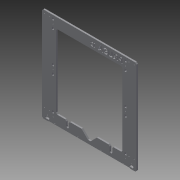
# Autodesk Inventor part: Main_frame_import
Saved by Autodesk Inventor 2015 (Build 190159000, 159)
## iProperties
Created: 2015-04-20
Part Number: Main_frame_import
Material: Generic
Document SubType Name: Modeling
Designer: X
Density: 1 g/cm^3
Appearance: Default
Author: X
Autodesk Inventor part; units mm, degrees
(part 1 of 2)
ref_plane "YZ Plane" through (0, 0, 0) normal (1, 0, 0) x (0, 1, 0)
ref_plane "XZ Plane" through (0, 0, 0) normal (0, 1, 0) x (-1, 0, 0)
ref_plane "XY Plane" through (0, 0, 0) normal (0, 0, 1) x (1, 0, 0)
sketch "Sketch1" plane through (0, 0, 0) normal (0, 1, 0) x (-1, 0, 0)
  line L0 (-246.1714, 171.3681) -> (-245.3714, 170.9681)
  line L1 (-245.3714, 170.9681) -> (-244.7714, 170.3681)
  line L2 (-244.7714, 170.3681) -> (-244.4714, 169.7681)
  line L3 (-244.4714, 169.7681) -> (-244.2714, 168.9681)
  line L4 (-244.2714, 168.9681) -> (-244.3714, 168.0681)
  line L5 (-244.3714, 168.0681) -> (-244.7714, 167.2681)
  line L6 (-244.7714, 167.2681) -> (-245.2714, 166.6681)
  line L7 (-245.2714, 166.6681) -> (-246.1714, 166.1681)
  line L8 (-246.1714, 166.1681) -> (-247.0714, 165.9681)
  line L9 (-247.0714, 165.9681) -> (-249.9714, 165.9681)
  line L10 (-249.9714, 165.9681) -> (-249.9714, 162.5681)
  line L11 (-249.9714, 162.5681) -> (-247.0714, 162.5681)
  line L12 (-247.0714, 162.5681) -> (-245.3714, 162.6681)
  line L13 (-245.3714, 162.6681) -> (-243.3714, 163.2681)
  line L14 (-243.3714, 163.2681) -> (-241.8714, 164.2681)
  line L15 (-241.8714, 164.2681) -> (-240.9714, 165.3681)
  line L16 (-240.9714, 165.3681) -> (-240.3714, 166.6681)
  line L17 (-240.3714, 166.6681) -> (-240.1714, 167.9681)
  line L18 (-240.1714, 167.9681) -> (-240.1714, 169.6681)
  line L19 (-240.1714, 169.6681) -> (-240.4714, 171.1681)
  line L20 (-240.4714, 171.1681) -> (-241.1714, 172.4681)
  line L21 (-241.1714, 172.4681) -> (-241.9714, 173.4681)
  line L22 (-241.9714, 173.4681) -> (-243.2714, 174.3681)
  line L23 (-243.2714, 174.3681) -> (-244.1714, 174.6681)
  line L24 (-244.1714, 174.6681) -> (-245.6714, 174.8681)
  line L25 (-245.6714, 174.8681) -> (-247.0714, 174.9681)
  line L26 (-247.0714, 174.9681) -> (-255.4714, 174.9681)
  line L27 (-255.4714, 174.9681) -> (-255.4714, 154.9681)
  line L28 (-255.4714, 154.9681) -> (-251.4714, 154.9681)
  line L29 (-251.4714, 154.9681) -> (-251.4714, 171.5681)
  line L30 (-251.4714, 171.5681) -> (-247.1714, 171.5681)
  line L31 (-247.1714, 171.5681) -> (-246.1714, 171.3681)
  line L32 (-164.1977, 155.0432) -> (-165.9232, 159.56)
  line L33 (-165.9232, 159.56) -> (-172.7744, 159.56)
  line L34 (-172.7744, 159.56) -> (-171.6072, 162.8587)
  line L35 (-171.6072, 162.8587) -> (-167.2427, 162.9094)
  line L36 (-167.2427, 162.9094) -> (-170.034, 170.2174)
  line L37 (-170.034, 170.2174) -> (-175.5657, 154.9417)
  line L38 (-175.5657, 154.9417) -> (-179.9302, 154.9417)
  line L39 (-179.9302, 154.9417) -> (-172.064, 174.8864)
  line L40 (-172.064, 174.8864) -> (-167.801, 174.8864)
  line L41 (-167.801, 174.8864) -> (-159.884, 154.9925)
  line L42 (-159.884, 154.9925) -> (-164.1977, 155.0432)
  line L43 (-213.334, 155.5625) -> (-211.5964, 154.9262)
  line L44 (-211.5964, 154.9262) -> (-208.9776, 154.5835)
  line L45 (-208.9776, 154.5835) -> (-206.3589, 154.7793)
  line L46 (-206.3589, 154.7793) -> (-204.2541, 155.4401)
  line L47 (-204.2541, 155.4401) -> (-202.9325, 156.2967)
  line L48 (-202.9325, 156.2967) -> (-201.7822, 157.4225)
  line L49 (-201.7822, 157.4225) -> (-201.0479, 159.4683)
  line L50 (-201.0479, 159.4683) -> (-200.7053, 162.2339)
  line L51 (-200.7053, 162.2339) -> (-200.7053, 166.1498)
  line L52 (-200.7053, 166.1498) -> (-200.7298, 174.9605)
  line L53 (-200.7298, 174.9605) -> (-204.7925, 174.9605)
  line L54 (-204.7925, 174.9605) -> (-204.768, 163.0171)
  line L55 (-204.768, 163.0171) -> (-204.8904, 161.3039)
  line L56 (-204.8904, 161.3039) -> (-205.2575, 159.5662)
  line L57 (-205.2575, 159.5662) -> (-206.1631, 158.6851)
  line L58 (-206.1631, 158.6851) -> (-207.3623, 158.1712)
  line L59 (-207.3623, 158.1712) -> (-208.8063, 158.0733)
  line L60 (-208.8063, 158.0733) -> (-210.2992, 158.318)
  line L61 (-210.2992, 158.318) -> (-211.5229, 159.0523)
  line L62 (-211.5229, 159.0523) -> (-212.3306, 160.276)
  line L63 (-212.3306, 160.276) -> (-212.6488, 162.185)
  line L64 (-212.6488, 162.185) -> (-212.6243, 170.1391)
  line L65 (-212.6243, 170.1391) -> (-212.6243, 174.9605)
  line L66 (-212.6243, 174.9605) -> (-216.6714, 174.9681)
  line L67 (-216.6714, 174.9681) -> (-216.7115, 163.9816)
  line L68 (-216.7115, 163.9816) -> (-216.4912, 160.3594)
  line L69 (-216.4912, 160.3594) -> (-216.0996, 158.6952)
  line L70 (-216.0996, 158.6952) -> (-215.5122, 157.496)
  line L71 (-215.5122, 157.496) -> (-214.5822, 156.3946)
  line L72 (-214.5822, 156.3946) -> (-213.334, 155.5625)
  line L73 (-224.6714, 174.3681) -> (-225.5714, 174.6681)
  line L74 (-225.5714, 174.6681) -> (-227.0714, 174.8681)
  line L75 (-227.0714, 174.8681) -> (-228.4714, 174.9681)
  line L76 (-228.4714, 174.9681) -> (-236.8714, 174.9681)
  line L77 (-236.8714, 174.9681) -> (-236.8714, 154.9681)
  line L78 (-236.8714, 154.9681) -> (-232.8714, 154.9681)
  line L79 (-232.8714, 154.9681) -> (-232.8714, 171.5681)
  line L80 (-232.8714, 171.5681) -> (-228.5714, 171.5681)
  line L81 (-228.5714, 171.5681) -> (-227.5714, 171.3681)
  line L82 (-227.5714, 171.3681) -> (-226.7714, 170.9681)
  line L83 (-226.7714, 170.9681) -> (-226.1714, 170.3681)
  line L84 (-226.1714, 170.3681) -> (-225.8714, 169.7681)
  line L85 (-225.8714, 169.7681) -> (-225.6714, 168.9681)
  line L86 (-225.6714, 168.9681) -> (-225.7714, 168.0681)
  line L87 (-225.7714, 168.0681) -> (-226.1714, 167.2681)
  line L88 (-226.1714, 167.2681) -> (-226.6714, 166.6681)
  line L89 (-226.6714, 166.6681) -> (-227.5714, 166.1681)
  line L90 (-227.5714, 166.1681) -> (-228.4714, 165.9681)
  line L91 (-228.4714, 165.9681) -> (-231.3714, 165.9681)
  line L92 (-231.3714, 165.9681) -> (-231.3714, 162.5681)
  line L93 (-231.3714, 162.5681) -> (-228.9774, 162.5681)
  line L94 (-228.9774, 162.5681) -> (-223.7358, 154.972)
  line L95 (-223.7358, 154.972) -> (-218.8614, 154.972)
  line L96 (-218.8614, 154.972) -> (-223.0424, 161.6209)
  line L97 (-223.0424, 161.6209) -> (-224.001, 162.5794)
  line L98 (-224.001, 162.5794) -> (-224.7714, 163.2681)
  line L99 (-224.7714, 163.2681) -> (-223.2714, 164.2681)
  line L100 (-223.2714, 164.2681) -> (-222.3714, 165.3681)
  line L101 (-222.3714, 165.3681) -> (-221.7714, 166.6681)
  line L102 (-221.7714, 166.6681) -> (-221.5714, 167.9681)
  line L103 (-221.5714, 167.9681) -> (-221.5714, 169.6681)
  line L104 (-221.5714, 169.6681) -> (-221.8714, 171.1681)
  line L105 (-221.8714, 171.1681) -> (-222.5714, 172.4681)
  line L106 (-222.5714, 172.4681) -> (-223.3714, 173.4681)
  line L107 (-223.3714, 173.4681) -> (-224.6714, 174.3681)
  line L108 (-186.6292, 166.8679) -> (-190.1817, 167.7814)
  line L109 (-190.1817, 167.7814) -> (-192.5162, 168.7964)
  line L110 (-192.5162, 168.7964) -> (-192.8207, 169.7099)
  line L111 (-192.8207, 169.7099) -> (-192.8153, 170.4712)
  line L112 (-192.8153, 170.4712) -> (-192.3453, 171.176)
  line L113 (-192.3453, 171.176) -> (-191.4936, 171.6753)
  line L114 (-191.4936, 171.6753) -> (-190.4657, 171.9396)
  line L115 (-190.4657, 171.9396) -> (-189.0854, 171.9984)
  line L116 (-189.0854, 171.9984) -> (-187.7931, 171.7928)
  line L117 (-187.7931, 171.7928) -> (-186.6477, 171.1467)
  line L118 (-186.6477, 171.1467) -> (-186.1191, 170.295)
  line L119 (-186.1191, 170.295) -> (-185.8254, 169.0027)
  line L120 (-185.8254, 169.0027) -> (-181.7572, 169.2532)
  line L121 (-181.7572, 169.2532) -> (-182.1632, 171.2324)
  line L122 (-182.1632, 171.2324) -> (-183.2797, 173.2117)
  line L123 (-183.2797, 173.2117) -> (-184.8529, 174.3282)
  line L124 (-184.8529, 174.3282) -> (-186.8829, 175.0894)
  line L125 (-186.8829, 175.0894) -> (-189.0144, 175.2417)
  line L126 (-189.0144, 175.2417) -> (-190.6892, 175.2417)
  line L127 (-190.6892, 175.2417) -> (-193.3282, 174.6327)
  line L128 (-193.3282, 174.6327) -> (-195.2059, 173.4654)
  line L129 (-195.2059, 173.4654) -> (-196.4239, 171.6384)
  line L130 (-196.4239, 171.6384) -> (-196.8299, 170.3189)
  line L131 (-196.8299, 170.3189) -> (-196.6269, 168.3397)
  line L132 (-196.6269, 168.3397) -> (-195.8149, 166.5634)
  line L133 (-195.8149, 166.5634) -> (-194.3939, 165.2947)
  line L134 (-194.3939, 165.2947) -> (-191.5519, 164.0259)
  line L135 (-191.5519, 164.0259) -> (-186.9844, 162.9094)
  line L136 (-186.9844, 162.9094) -> (-185.7157, 162.1482)
  line L137 (-185.7157, 162.1482) -> (-185.3604, 161.1332)
  line L138 (-185.3604, 161.1332) -> (-185.4112, 159.9659)
  line L139 (-185.4112, 159.9659) -> (-186.2232, 158.9002)
  line L140 (-186.2232, 158.9002) -> (-187.4412, 158.1897)
  line L141 (-187.4412, 158.1897) -> (-189.0652, 158.0375)
  line L142 (-189.0652, 158.0375) -> (-190.9937, 158.3927)
  line L143 (-190.9937, 158.3927) -> (-192.4654, 159.3062)
  line L144 (-192.4654, 159.3062) -> (-193.3789, 160.8794)
  line L145 (-193.3789, 160.8794) -> (-193.5819, 161.7422)
  line L146 (-193.5819, 161.7422) -> (-197.4896, 161.3869)
  line L147 (-197.4896, 161.3869) -> (-196.8806, 159.1032)
  line L148 (-196.8806, 159.1032) -> (-195.4089, 156.718)
  line L149 (-195.4089, 156.718) -> (-192.9222, 155.1955)
  line L150 (-192.9222, 155.1955) -> (-190.2832, 154.6372)
  line L151 (-190.2832, 154.6372) -> (-187.7457, 154.7387)
  line L152 (-187.7457, 154.7387) -> (-184.4469, 155.5507)
  line L153 (-184.4469, 155.5507) -> (-182.3154, 157.4285)
  line L154 (-182.3154, 157.4285) -> (-181.3004, 159.357)
  line L155 (-181.3004, 159.357) -> (-181.3004, 161.8944)
  line L156 (-181.3004, 161.8944) -> (-182.0109, 163.9244)
  line L157 (-182.0109, 163.9244) -> (-183.6349, 165.7007)
  line L158 (-183.6349, 165.7007) -> (-186.6292, 166.8679)
  line L159 (7.7286, -179.0318) -> (7.7899, -179.4977)
  line L160 (7.7899, -179.4977) -> (7.9698, -179.9318)
  line L161 (7.9698, -179.9318) -> (8.2558, -180.3046)
  line L162 (8.2558, -180.3046) -> (8.6286, -180.5907)
  line L163 (8.6286, -180.5907) -> (9.0627, -180.7705)
  line L164 (9.0627, -180.7705) -> (9.5286, -180.8318)
  line L165 (9.5286, -180.8318) -> (9.9945, -180.7705)
  line L166 (9.9945, -180.7705) -> (10.4286, -180.5907)
  line L167 (10.4286, -180.5907) -> (10.8014, -180.3046)
  line L168 (10.8014, -180.3046) -> (11.0875, -179.9318)
  line L169 (11.0875, -179.9318) -> (11.2673, -179.4977)
  line L170 (11.2673, -179.4977) -> (11.3286, -179.0318)
  line L171 (11.3286, -179.0318) -> (11.2673, -178.566)
  line L172 (11.2673, -178.566) -> (11.0875, -178.1318)
  line L173 (11.0875, -178.1318) -> (10.8014, -177.759)
  line L174 (10.8014, -177.759) -> (10.4286, -177.473)
  line L175 (10.4286, -177.473) -> (9.9945, -177.2932)
  line L176 (9.9945, -177.2932) -> (9.5286, -177.2318)
  line L177 (9.5286, -177.2318) -> (9.0627, -177.2932)
  line L178 (9.0627, -177.2932) -> (8.6286, -177.473)
  line L179 (8.6286, -177.473) -> (8.2558, -177.759)
  line L180 (8.2558, -177.759) -> (7.9698, -178.1318)
  line L181 (7.9698, -178.1318) -> (7.7899, -178.566)
  line L182 (7.7899, -178.566) -> (7.7286, -179.0318)
  line L183 (-78.6714, -179.0318) -> (-78.7327, -178.566)
  line L184 (-78.7327, -178.566) -> (-78.9125, -178.1318)
  line L185 (-78.9125, -178.1318) -> (-79.1986, -177.759)
  line L186 (-79.1986, -177.759) -> (-79.5714, -177.473)
  line L187 (-79.5714, -177.473) -> (-80.0055, -177.2932)
  line L188 (-80.0055, -177.2932) -> (-80.4714, -177.2318)
  line L189 (-80.4714, -177.2318) -> (-80.9373, -177.2932)
  line L190 (-80.9373, -177.2932) -> (-81.3714, -177.473)
  line L191 (-81.3714, -177.473) -> (-81.7442, -177.759)
  line L192 (-81.7442, -177.759) -> (-82.0302, -178.1318)
  line L193 (-82.0302, -178.1318) -> (-82.21, -178.566)
  line L194 (-82.21, -178.566) -> (-82.2714, -179.0318)
  line L195 (-82.2714, -179.0318) -> (-82.21, -179.4977)
  line L196 (-82.21, -179.4977) -> (-82.0302, -179.9318)
  line L197 (-82.0302, -179.9318) -> (-81.7442, -180.3046)
  line L198 (-81.7442, -180.3046) -> (-81.3714, -180.5907)
  line L199 (-81.3714, -180.5907) -> (-80.9373, -180.7705)
  line L200 (-80.9373, -180.7705) -> (-80.4714, -180.8318)
  line L201 (-80.4714, -180.8318) -> (-80.0055, -180.7705)
  line L202 (-80.0055, -180.7705) -> (-79.5714, -180.5907)
  line L203 (-79.5714, -180.5907) -> (-79.1986, -180.3046)
  line L204 (-79.1986, -180.3046) -> (-78.9125, -179.9318)
  line L205 (-78.9125, -179.9318) -> (-78.7327, -179.4977)
  line L206 (-78.7327, -179.4977) -> (-78.6714, -179.0318)
  line L207 (-168.6714, -179.0318) -> (-168.7327, -178.566)
  line L208 (-168.7327, -178.566) -> (-168.9125, -178.1318)
  line L209 (-168.9125, -178.1318) -> (-169.1986, -177.759)
  line L210 (-169.1986, -177.759) -> (-169.5714, -177.473)
  line L211 (-169.5714, -177.473) -> (-170.0055, -177.2932)
  line L212 (-170.0055, -177.2932) -> (-170.4714, -177.2318)
  line L213 (-170.4714, -177.2318) -> (-170.9372, -177.2932)
  line L214 (-170.9372, -177.2932) -> (-171.3714, -177.473)
  line L215 (-171.3714, -177.473) -> (-171.7442, -177.759)
  line L216 (-171.7442, -177.759) -> (-172.0302, -178.1318)
  line L217 (-172.0302, -178.1318) -> (-172.21, -178.566)
  line L218 (-172.21, -178.566) -> (-172.2714, -179.0318)
  line L219 (-172.2714, -179.0318) -> (-172.21, -179.4977)
  line L220 (-172.21, -179.4977) -> (-172.0302, -179.9318)
  line L221 (-172.0302, -179.9318) -> (-171.7442, -180.3046)
  line L222 (-171.7442, -180.3046) -> (-171.3714, -180.5907)
  line L223 (-171.3714, -180.5907) -> (-170.9372, -180.7705)
  line L224 (-170.9372, -180.7705) -> (-170.4714, -180.8318)
  line L225 (-170.4714, -180.8318) -> (-170.0055, -180.7705)
  line L226 (-170.0055, -180.7705) -> (-169.5714, -180.5907)
  line L227 (-169.5714, -180.5907) -> (-169.1986, -180.3046)
  line L228 (-169.1986, -180.3046) -> (-168.9125, -179.9318)
  line L229 (-168.9125, -179.9318) -> (-168.7327, -179.4977)
  line L230 (-168.7327, -179.4977) -> (-168.6714, -179.0318)
  line L231 (-258.6714, -179.0318) -> (-258.7327, -178.566)
  line L232 (-258.7327, -178.566) -> (-258.9125, -178.1318)
  line L233 (-258.9125, -178.1318) -> (-259.1986, -177.759)
  line L234 (-259.1986, -177.759) -> (-259.5714, -177.473)
  line L235 (-259.5714, -177.473) -> (-260.0055, -177.2932)
  line L236 (-260.0055, -177.2932) -> (-260.4714, -177.2318)
  line L237 (-260.4714, -177.2318) -> (-260.9372, -177.2932)
  line L238 (-260.9372, -177.2932) -> (-261.3714, -177.473)
  line L239 (-261.3714, -177.473) -> (-261.7442, -177.759)
  line L240 (-261.7442, -177.759) -> (-262.0302, -178.1318)
  line L241 (-262.0302, -178.1318) -> (-262.21, -178.566)
  line L242 (-262.21, -178.566) -> (-262.2714, -179.0318)
  line L243 (-262.2714, -179.0318) -> (-262.21, -179.4977)
  line L244 (-262.21, -179.4977) -> (-262.0302, -179.9318)
  line L245 (-262.0302, -179.9318) -> (-261.7442, -180.3046)
  line L246 (-261.7442, -180.3046) -> (-261.3714, -180.5907)
  line L247 (-261.3714, -180.5907) -> (-260.9372, -180.7705)
  line L248 (-260.9372, -180.7705) -> (-260.4714, -180.8318)
  line L249 (-260.4714, -180.8318) -> (-260.0055, -180.7705)
  line L250 (-260.0055, -180.7705) -> (-259.5714, -180.5907)
  line L251 (-259.5714, -180.5907) -> (-259.1986, -180.3046)
  line L252 (-259.1986, -180.3046) -> (-258.9125, -179.9318)
  line L253 (-258.9125, -179.9318) -> (-258.7327, -179.4977)
  line L254 (-258.7327, -179.4977) -> (-258.6714, -179.0318)
  line L255 (-129.2375, 159.816) -> (-129.3394, 158.7675)
  line L256 (-129.3394, 158.7675) -> (-129.6449, 157.8145)
  line L257 (-129.6449, 157.8145) -> (-130.1465, 156.9772)
  line L258 (-130.1465, 156.9772) -> (-130.8367, 156.2757)
  line L259 (-130.8367, 156.2757) -> (-131.7004, 155.7162)
  line L260 (-131.7004, 155.7162) -> (-132.7025, 155.3051)
  line L261 (-132.7025, 155.3051) -> (-133.8905, 155.0524)
  line L262 (-133.8905, 155.0524) -> (-135.3125, 154.9681)
  line L263 (-135.3125, 154.9681) -> (-136.9381, 155.0411)
  line L264 (-136.9381, 155.0411) -> (-138.3147, 155.2598)
  line L265 (-138.3147, 155.2598) -> (-140.3515, 155.9136)
  line L266 (-140.3515, 155.9136) -> (-140.3515, 159.1623)
  line L267 (-140.3515, 159.1623) -> (-139.9894, 159.1623)
  line L268 (-139.9894, 159.1623) -> (-139.093, 158.6745)
  line L269 (-139.093, 158.6745) -> (-138.0532, 158.2571)
  line L270 (-138.0532, 158.2571) -> (-136.9909, 157.9704)
  line L271 (-136.9909, 157.9704) -> (-136.0266, 157.8749)
  line L272 (-136.0266, 157.8749) -> (-134.8448, 157.9704)
  line L273 (-134.8448, 157.9704) -> (-134.2577, 158.1225)
  line L274 (-134.2577, 158.1225) -> (-133.7736, 158.3878)
  line L275 (-133.7736, 158.3878) -> (-133.2255, 159.0064)
  line L276 (-133.2255, 159.0064) -> (-133.0708, 159.4502)
  line L277 (-133.0708, 159.4502) -> (-133.0193, 160.0474)
  line L278 (-133.0193, 160.0474) -> (-133.0922, 160.6345)
  line L279 (-133.0922, 160.6345) -> (-133.311, 161.0682)
  line L280 (-133.311, 161.0682) -> (-133.6504, 161.3763)
  line L281 (-133.6504, 161.3763) -> (-134.0854, 161.5862)
  line L282 (-134.0854, 161.5862) -> (-135.2421, 161.7773)
  line L283 (-135.2421, 161.7773) -> (-136.4289, 161.7974)
  line L284 (-136.4289, 161.7974) -> (-137.0726, 161.7974)
  line L285 (-137.0726, 161.7974) -> (-137.0726, 164.4326)
  line L286 (-137.0726, 164.4326) -> (-136.4792, 164.4326)
  line L287 (-136.4792, 164.4326) -> (-135.222, 164.4929)
  line L288 (-135.222, 164.4929) -> (-134.2463, 164.7343)
  line L289 (-134.2463, 164.7343) -> (-133.6177, 165.2674)
  line L290 (-133.6177, 165.2674) -> (-133.448, 165.6697)
  line L291 (-133.448, 165.6697) -> (-133.3914, 166.1927)
  line L292 (-133.3914, 166.1927) -> (-133.4442, 166.6038)
  line L293 (-133.4442, 166.6038) -> (-133.6026, 166.932)
  line L294 (-133.6026, 166.932) -> (-134.1256, 167.3795)
  line L295 (-134.1256, 167.3795) -> (-134.9705, 167.6209)
  line L296 (-134.9705, 167.6209) -> (-135.7953, 167.6813)
  line L297 (-135.7953, 167.6813) -> (-136.9217, 167.5505)
  line L298 (-136.9217, 167.5505) -> (-138.0382, 167.2186)
  line L299 (-138.0382, 167.2186) -> (-138.9232, 166.8012)
  line L300 (-138.9232, 166.8012) -> (-139.6072, 166.414)
  line L301 (-139.6072, 166.414) -> (-139.919, 166.414)
  line L302 (-139.919, 166.414) -> (-139.919, 169.6224)
  line L303 (-139.919, 169.6224) -> (-137.832, 170.2611)
  line L304 (-137.832, 170.2611) -> (-136.5056, 170.4912)
  line L305 (-136.5056, 170.4912) -> (-135.1515, 170.5679)
  line L306 (-135.1515, 170.5679) -> (-133.9031, 170.51)
  line L307 (-133.9031, 170.51) -> (-132.8332, 170.3365)
  line L308 (-132.8332, 170.3365) -> (-131.9242, 170.0524)
  line L309 (-131.9242, 170.0524) -> (-131.1586, 169.6627)
  line L310 (-131.1586, 169.6627) -> (-130.4897, 169.1258)
  line L311 (-130.4897, 169.1258) -> (-130.012, 168.4608)
  line L312 (-130.012, 168.4608) -> (-129.7253, 167.685)
  line L313 (-129.7253, 167.685) -> (-129.6298, 166.8163)
  line L314 (-129.6298, 166.8163) -> (-129.8146, 165.6182)
  line L315 (-129.8146, 165.6182) -> (-130.369, 164.5784)
  line L316 (-130.369, 164.5784) -> (-131.2252, 163.7876)
  line L317 (-131.2252, 163.7876) -> (-132.3152, 163.3363)
  line L318 (-132.3152, 163.3363) -> (-132.3152, 163.1955)
  line L319 (-132.3152, 163.1955) -> (-131.2742, 162.9239)
  line L320 (-131.2742, 162.9239) -> (-130.2835, 162.3003)
  line L321 (-130.2835, 162.3003) -> (-129.8699, 161.8515)
  line L322 (-129.8699, 161.8515) -> (-129.5342, 161.2895)
  line L323 (-129.5342, 161.2895) -> (-129.3117, 160.6119)
  line L324 (-129.3117, 160.6119) -> (-129.2375, 159.816)
  line L325 (-142.6346, 167.8724) -> (-146.356, 167.8724)
  line L326 (-146.356, 167.8724) -> (-146.356, 170.6182)
  line L327 (-146.356, 170.6182) -> (-142.6346, 170.6182)
  line L328 (-142.6346, 170.6182) -> (-142.6346, 167.8724)
  line L329 (-142.7352, 154.9681) -> (-146.2554, 154.9681)
  line L330 (-146.2554, 154.9681) -> (-146.2554, 166.2631)
  line L331 (-146.2554, 166.2631) -> (-142.7352, 166.2631)
  line L332 (-142.7352, 166.2631) -> (-142.7352, 154.9681)
  line L333 (-266.9805, 156.7019) -> (-267.4464, 156.7632)
  line L334 (-267.4464, 156.7632) -> (-267.9123, 156.7018)
  line L335 (-267.9123, 156.7018) -> (-268.3464, 156.5219)
  line L336 (-268.3464, 156.5219) -> (-268.7191, 156.2358)
  line L337 (-268.7191, 156.2358) -> (-269.0051, 155.863)
  line L338 (-269.0051, 155.863) -> (-269.1849, 155.4288)
  line L339 (-269.1849, 155.4288) -> (-269.2461, 154.9629)
  line L340 (-269.2461, 154.9629) -> (-269.1847, 154.4971)
  line L341 (-269.1847, 154.4971) -> (-269.0048, 154.063)
  line L342 (-269.0048, 154.063) -> (-268.7187, 153.6902)
  line L343 (-268.7187, 153.6902) -> (-268.3459, 153.4042)
  line L344 (-268.3459, 153.4042) -> (-267.9118, 153.2244)
  line L345 (-267.9118, 153.2244) -> (-267.4459, 153.1632)
  line L346 (-267.4459, 153.1632) -> (-266.98, 153.2246)
  line L347 (-266.98, 153.2246) -> (-266.5459, 153.4045)
  line L348 (-266.5459, 153.4045) -> (-266.1732, 153.6906)
  line L349 (-266.1732, 153.6906) -> (-265.8872, 154.0634)
  line L350 (-265.8872, 154.0634) -> (-265.7074, 154.4976)
  line L351 (-265.7074, 154.4976) -> (-265.6461, 154.9634)
  line L352 (-265.6461, 154.9634) -> (-265.7075, 155.4293)
  line L353 (-265.7075, 155.4293) -> (-265.8874, 155.8634)
  line L354 (-265.8874, 155.8634) -> (-266.1735, 156.2362)
  line L355 (-266.1735, 156.2362) -> (-266.5464, 156.5222)
  line L356 (-266.5464, 156.5222) -> (-266.9805, 156.7019)
  line L357 (-281.7214, 176.2542) -> (-282.0074, 175.8814)
  line L358 (-282.0074, 175.8814) -> (-282.1872, 175.4473)
  line L359 (-282.1872, 175.4473) -> (-282.2485, 174.9814)
  line L360 (-282.2485, 174.9814) -> (-282.1871, 174.5155)
  line L361 (-282.1871, 174.5155) -> (-282.0072, 174.0814)
  line L362 (-282.0072, 174.0814) -> (-281.7211, 173.7087)
  line L363 (-281.7211, 173.7087) -> (-281.3482, 173.4227)
  line L364 (-281.3482, 173.4227) -> (-280.9141, 173.2429)
  line L365 (-280.9141, 173.2429) -> (-280.4482, 173.1816)
  line L366 (-280.4482, 173.1816) -> (-279.9823, 173.243)
  line L367 (-279.9823, 173.243) -> (-279.5482, 173.4229)
  line L368 (-279.5482, 173.4229) -> (-279.1755, 173.709)
  line L369 (-279.1755, 173.709) -> (-278.8895, 174.0818)
  line L370 (-278.8895, 174.0818) -> (-278.7097, 174.516)
  line L371 (-278.7097, 174.516) -> (-278.6485, 174.9819)
  line L372 (-278.6485, 174.9819) -> (-278.7099, 175.4477)
  line L373 (-278.7099, 175.4477) -> (-278.8897, 175.8818)
  line L374 (-278.8897, 175.8818) -> (-279.1759, 176.2546)
  line L375 (-279.1759, 176.2546) -> (-279.5487, 176.5406)
  line L376 (-279.5487, 176.5406) -> (-279.9828, 176.7204)
  line L377 (-279.9828, 176.7204) -> (-280.4487, 176.7816)
  line L378 (-280.4487, 176.7816) -> (-280.9146, 176.7202)
  line L379 (-280.9146, 176.7202) -> (-281.3487, 176.5403)
  line L380 (-281.3487, 176.5403) -> (-281.7214, 176.2542)
  line L381 (-300.4667, 173.1816) -> (-300.0008, 173.243)
  line L382 (-300.0008, 173.243) -> (-299.5667, 173.4229)
  line L383 (-299.5667, 173.4229) -> (-299.1939, 173.709)
  line L384 (-299.1939, 173.709) -> (-298.9079, 174.0818)
  line L385 (-298.9079, 174.0818) -> (-298.7282, 174.516)
  line L386 (-298.7282, 174.516) -> (-298.6669, 174.9819)
  line L387 (-298.6669, 174.9819) -> (-298.7283, 175.4477)
  line L388 (-298.7283, 175.4477) -> (-298.9082, 175.8818)
  line L389 (-298.9082, 175.8818) -> (-299.1943, 176.2546)
  line L390 (-299.1943, 176.2546) -> (-299.5671, 176.5406)
  line L391 (-299.5671, 176.5406) -> (-300.0013, 176.7204)
  line L392 (-300.0013, 176.7204) -> (-300.4672, 176.7816)
  line L393 (-300.4672, 176.7816) -> (-300.933, 176.7202)
  line L394 (-300.933, 176.7202) -> (-301.3671, 176.5403)
  line L395 (-301.3671, 176.5403) -> (-301.7399, 176.2542)
  line L396 (-301.7399, 176.2542) -> (-302.0259, 175.8814)
  line L397 (-302.0259, 175.8814) -> (-302.2056, 175.4473)
  line L398 (-302.2056, 175.4473) -> (-302.2669, 174.9814)
  line L399 (-302.2669, 174.9814) -> (-302.2055, 174.5155)
  line L400 (-302.2055, 174.5155) -> (-302.0256, 174.0814)
  line L401 (-302.0256, 174.0814) -> (-301.7395, 173.7087)
  line L402 (-301.7395, 173.7087) -> (-301.3667, 173.4227)
  line L403 (-301.3667, 173.4227) -> (-300.9325, 173.2429)
  line L404 (-300.9325, 173.2429) -> (-300.4667, 173.1816)
  line L405 (-265.6461, -0.0347) -> (-265.7075, 0.4312)
  line L406 (-265.7075, 0.4312) -> (-265.8874, 0.8653)
  line L407 (-265.8874, 0.8653) -> (-266.1735, 1.238)
  line L408 (-266.1735, 1.238) -> (-266.5464, 1.524)
  line L409 (-266.5464, 1.524) -> (-266.9805, 1.7038)
  line L410 (-266.9805, 1.7038) -> (-267.4464, 1.765)
  line L411 (-267.4464, 1.765) -> (-267.9123, 1.7036)
  line L412 (-267.9123, 1.7036) -> (-268.3464, 1.5237)
  line L413 (-268.3464, 1.5237) -> (-268.7191, 1.2376)
  line L414 (-268.7191, 1.2376) -> (-269.0051, 0.8648)
  line L415 (-269.0051, 0.8648) -> (-269.1849, 0.4307)
  line L416 (-269.1849, 0.4307) -> (-269.2461, -0.0352)
  line L417 (-269.2461, -0.0352) -> (-269.1847, -0.5011)
  line L418 (-269.1847, -0.5011) -> (-269.0048, -0.9352)
  line L419 (-269.0048, -0.9352) -> (-268.7187, -1.3079)
  line L420 (-268.7187, -1.3079) -> (-268.3459, -1.5939)
  line L421 (-268.3459, -1.5939) -> (-267.9118, -1.7737)
  line L422 (-267.9118, -1.7737) -> (-267.4459, -1.835)
  line L423 (-267.4459, -1.835) -> (-266.98, -1.7736)
  line L424 (-266.98, -1.7736) -> (-266.5459, -1.5937)
  line L425 (-266.5459, -1.5937) -> (-266.1732, -1.3076)
  line L426 (-266.1732, -1.3076) -> (-265.8872, -0.9347)
  line L427 (-265.8872, -0.9347) -> (-265.7074, -0.5006)
  line L428 (-265.7074, -0.5006) -> (-265.6461, -0.0347)
  line L429 (-266.5884, -158.4625) -> (-267.0226, -158.2828)
  line L430 (-267.0226, -158.2828) -> (-267.4884, -158.2215)
  line L431 (-267.4884, -158.2215) -> (-267.9543, -158.2829)
  line L432 (-267.9543, -158.2829) -> (-268.3884, -158.4628)
  line L433 (-268.3884, -158.4628) -> (-268.7611, -158.7489)
  line L434 (-268.7611, -158.7489) -> (-269.0472, -159.1217)
  line L435 (-269.0472, -159.1217) -> (-269.2269, -159.5559)
  line L436 (-269.2269, -159.5559) -> (-269.2882, -160.0218)
  line L437 (-269.2882, -160.0218) -> (-269.2268, -160.4876)
  line L438 (-269.2268, -160.4876) -> (-269.0469, -160.9217)
  line L439 (-269.0469, -160.9217) -> (-268.7608, -161.2945)
  line L440 (-268.7608, -161.2945) -> (-268.388, -161.5805)
  line L441 (-268.388, -161.5805) -> (-267.9538, -161.7603)
  line L442 (-267.9538, -161.7603) -> (-267.4879, -161.8215)
  line L443 (-267.4879, -161.8215) -> (-267.0221, -161.7601)
  line L444 (-267.0221, -161.7601) -> (-266.588, -161.5802)
  line L445 (-266.588, -161.5802) -> (-266.2152, -161.2941)
  line L446 (-266.2152, -161.2941) -> (-265.9292, -160.9213)
  line L447 (-265.9292, -160.9213) -> (-265.7494, -160.4871)
  line L448 (-265.7494, -160.4871) -> (-265.6882, -160.0213)
  line L449 (-265.6882, -160.0213) -> (-265.7496, -159.5554)
  line L450 (-265.7496, -159.5554) -> (-265.9295, -159.1213)
  line L451 (-265.9295, -159.1213) -> (-266.2156, -158.7485)
  line L452 (-266.2156, -158.7485) -> (-266.5884, -158.4625)
  line L453 (-292.0545, -164.1252) -> (-292.2343, -164.5594)
  line L454 (-292.2343, -164.5594) -> (-292.2955, -165.0252)
  line L455 (-292.2955, -165.0252) -> (-292.2341, -165.4911)
  line L456 (-292.2341, -165.4911) -> (-292.0543, -165.9252)
  line L457 (-292.0543, -165.9252) -> (-291.7682, -166.298)
  line L458 (-291.7682, -166.298) -> (-291.3953, -166.584)
  line L459 (-291.3953, -166.584) -> (-290.9612, -166.7637)
  line L460 (-290.9612, -166.7637) -> (-290.4953, -166.825)
  line L461 (-290.4953, -166.825) -> (-290.0294, -166.7636)
  line L462 (-290.0294, -166.7636) -> (-289.5953, -166.5837)
  line L463 (-289.5953, -166.5837) -> (-289.2226, -166.2976)
  line L464 (-289.2226, -166.2976) -> (-288.9366, -165.9248)
  line L465 (-288.9366, -165.9248) -> (-288.7568, -165.4906)
  line L466 (-288.7568, -165.4906) -> (-288.6955, -165.0247)
  line L467 (-288.6955, -165.0247) -> (-288.7569, -164.5589)
  line L468 (-288.7569, -164.5589) -> (-288.9368, -164.1248)
  line L469 (-288.9368, -164.1248) -> (-289.2229, -163.752)
  line L470 (-289.2229, -163.752) -> (-289.5958, -163.466)
  line L471 (-289.5958, -163.466) -> (-290.0299, -163.2863)
  line L472 (-290.0299, -163.2863) -> (-290.4958, -163.225)
  line L473 (-290.4958, -163.225) -> (-290.9617, -163.2864)
  line L474 (-290.9617, -163.2864) -> (-291.3958, -163.4663)
  line L475 (-291.3958, -163.4663) -> (-291.7685, -163.7524)
  line L476 (-291.7685, -163.7524) -> (-292.0545, -164.1252)
  line L477 (-278.6886, -145.0109) -> (-278.75, -144.545)
  line L478 (-278.75, -144.545) -> (-278.9299, -144.1109)
  line L479 (-278.9299, -144.1109) -> (-279.216, -143.7382)
  line L480 (-279.216, -143.7382) -> (-279.5888, -143.4522)
  line L481 (-279.5888, -143.4522) -> (-280.023, -143.2724)
  line L482 (-280.023, -143.2724) -> (-280.4889, -143.2111)
  line L483 (-280.4889, -143.2111) -> (-280.9547, -143.2725)
  line L484 (-280.9547, -143.2725) -> (-281.3888, -143.4524)
  line L485 (-281.3888, -143.4524) -> (-281.7616, -143.7385)
  line L486 (-281.7616, -143.7385) -> (-282.0476, -144.1114)
  line L487 (-282.0476, -144.1114) -> (-282.2274, -144.5455)
  line L488 (-282.2274, -144.5455) -> (-282.2886, -145.0114)
  line L489 (-282.2886, -145.0114) -> (-282.2272, -145.4773)
  line L490 (-282.2272, -145.4773) -> (-282.0473, -145.9114)
  line L491 (-282.0473, -145.9114) -> (-281.7612, -146.2841)
  line L492 (-281.7612, -146.2841) -> (-281.3884, -146.5701)
  line L493 (-281.3884, -146.5701) -> (-280.9542, -146.7499)
  line L494 (-280.9542, -146.7499) -> (-280.4884, -146.8111)
  line L495 (-280.4884, -146.8111) -> (-280.0225, -146.7497)
  line L496 (-280.0225, -146.7497) -> (-279.5884, -146.5699)
  line L497 (-279.5884, -146.5699) -> (-279.2156, -146.2838)
  line L498 (-279.2156, -146.2838) -> (-278.9296, -145.9109)
  line L499 (-278.9296, -145.9109) -> (-278.7499, -145.4768)
  line L500 (-278.7499, -145.4768) -> (-278.6886, -145.0109)
  line L501 (-299.2299, -143.7382) -> (-299.6027, -143.4522)
  line L502 (-299.6027, -143.4522) -> (-300.0368, -143.2724)
  line L503 (-300.0368, -143.2724) -> (-300.5027, -143.2111)
  line L504 (-300.5027, -143.2111) -> (-300.9686, -143.2725)
  line L505 (-300.9686, -143.2725) -> (-301.4027, -143.4524)
  line L506 (-301.4027, -143.4524) -> (-301.7754, -143.7385)
  line L507 (-301.7754, -143.7385) -> (-302.0614, -144.1114)
  line L508 (-302.0614, -144.1114) -> (-302.2412, -144.5455)
  line L509 (-302.2412, -144.5455) -> (-302.3025, -145.0114)
  line L510 (-302.3025, -145.0114) -> (-302.2411, -145.4773)
  line L511 (-302.2411, -145.4773) -> (-302.0612, -145.9114)
  line L512 (-302.0612, -145.9114) -> (-301.7751, -146.2841)
  line L513 (-301.7751, -146.2841) -> (-301.4022, -146.5701)
  line L514 (-301.4022, -146.5701) -> (-300.9681, -146.7499)
  line L515 (-300.9681, -146.7499) -> (-300.5022, -146.8111)
  line L516 (-300.5022, -146.8111) -> (-300.0363, -146.7497)
  line L517 (-300.0363, -146.7497) -> (-299.6022, -146.5699)
  line L518 (-299.6022, -146.5699) -> (-299.2295, -146.2838)
  line L519 (-299.2295, -146.2838) -> (-298.9435, -145.9109)
  line L520 (-298.9435, -145.9109) -> (-298.7637, -145.4768)
  line L521 (-298.7637, -145.4768) -> (-298.7025, -145.0109)
  line L522 (-298.7025, -145.0109) -> (-298.7639, -144.545)
  line L523 (-298.7639, -144.545) -> (-298.9437, -144.1109)
  line L524 (-298.9437, -144.1109) -> (-299.2299, -143.7382)
  line L525 (18.3279, -160.0318) -> (18.2666, -159.5661)
  line L526 (18.2666, -159.5661) -> (18.0868, -159.1322)
  line L527 (18.0868, -159.1322) -> (17.8009, -158.7595)
  line L528 (17.8009, -158.7595) -> (17.4283, -158.4736)
  line L529 (17.4283, -158.4736) -> (16.9943, -158.2939)
  line L530 (16.9943, -158.2939) -> (16.5286, -158.2325)
  line L531 (16.5286, -158.2325) -> (16.0629, -158.2939)
  line L532 (16.0629, -158.2939) -> (15.629, -158.4736)
  line L533 (15.629, -158.4736) -> (15.2563, -158.7595)
  line L534 (15.2563, -158.7595) -> (14.9704, -159.1322)
  line L535 (14.9704, -159.1322) -> (14.7906, -159.5661)
  line L536 (14.7906, -159.5661) -> (14.7293, -160.0318)
  line L537 (14.7293, -160.0318) -> (14.7906, -160.4975)
  line L538 (14.7906, -160.4975) -> (14.9704, -160.9315)
  line L539 (14.9704, -160.9315) -> (15.2563, -161.3041)
  line L540 (15.2563, -161.3041) -> (15.629, -161.59)
  line L541 (15.629, -161.59) -> (16.0629, -161.7698)
  line L542 (16.0629, -161.7698) -> (16.5286, -161.8311)
  line L543 (16.5286, -161.8311) -> (16.9943, -161.7698)
  line L544 (16.9943, -161.7698) -> (17.4283, -161.59)
  line L545 (17.4283, -161.59) -> (17.8009, -161.3041)
  line L546 (17.8009, -161.3041) -> (18.0868, -160.9315)
  line L547 (18.0868, -160.9315) -> (18.2666, -160.4975)
  line L548 (18.2666, -160.4975) -> (18.3279, -160.0318)
  line L549 (39.532, -163.2644) -> (39.0661, -163.3258)
  line L550 (39.0661, -163.3258) -> (38.632, -163.5057)
  line L551 (38.632, -163.5057) -> (38.2593, -163.7918)
  line L552 (38.2593, -163.7918) -> (37.9733, -164.1647)
  line L553 (37.9733, -164.1647) -> (37.7935, -164.5988)
  line L554 (37.7935, -164.5988) -> (37.7322, -165.0647)
  line L555 (37.7322, -165.0647) -> (37.7936, -165.5306)
  line L556 (37.7936, -165.5306) -> (37.9735, -165.9647)
  line L557 (37.9735, -165.9647) -> (38.2596, -166.3374)
  line L558 (38.2596, -166.3374) -> (38.6325, -166.6234)
  line L559 (38.6325, -166.6234) -> (39.0666, -166.8032)
  line L560 (39.0666, -166.8032) -> (39.5325, -166.8644)
  line L561 (39.5325, -166.8644) -> (39.9984, -166.803)
  line L562 (39.9984, -166.803) -> (40.4325, -166.6231)
  line L563 (40.4325, -166.6231) -> (40.8052, -166.337)
  line L564 (40.8052, -166.337) -> (41.0912, -165.9642)
  line L565 (41.0912, -165.9642) -> (41.271, -165.5301)
  line L566 (41.271, -165.5301) -> (41.3322, -165.0642)
  line L567 (41.3322, -165.0642) -> (41.2708, -164.5983)
  line L568 (41.2708, -164.5983) -> (41.091, -164.1642)
  line L569 (41.091, -164.1642) -> (40.8048, -163.7915)
  line L570 (40.8048, -163.7915) -> (40.432, -163.5055)
  line L571 (40.432, -163.5055) -> (39.9979, -163.3257)
  line L572 (39.9979, -163.3257) -> (39.532, -163.2644)
  line L573 (51.3217, -145.0853) -> (51.2603, -144.6195)
  line L574 (51.2603, -144.6195) -> (51.0804, -144.1854)
  line L575 (51.0804, -144.1854) -> (50.7943, -143.8126)
  line L576 (50.7943, -143.8126) -> (50.4214, -143.5266)
  line L577 (50.4214, -143.5266) -> (49.9873, -143.3469)
  line L578 (49.9873, -143.3469) -> (49.5214, -143.2856)
  line L579 (49.5214, -143.2856) -> (49.0555, -143.347)
  line L580 (49.0555, -143.347) -> (48.6214, -143.5269)
  line L581 (48.6214, -143.5269) -> (48.2487, -143.813)
  line L582 (48.2487, -143.813) -> (47.9627, -144.1858)
  line L583 (47.9627, -144.1858) -> (47.7829, -144.62)
  line L584 (47.7829, -144.62) -> (47.7217, -145.0858)
  line L585 (47.7217, -145.0858) -> (47.7831, -145.5517)
  line L586 (47.7831, -145.5517) -> (47.9629, -145.9858)
  line L587 (47.9629, -145.9858) -> (48.2491, -146.3586)
  line L588 (48.2491, -146.3586) -> (48.6219, -146.6446)
  line L589 (48.6219, -146.6446) -> (49.056, -146.8243)
  line L590 (49.056, -146.8243) -> (49.5219, -146.8856)
  line L591 (49.5219, -146.8856) -> (49.9878, -146.8242)
  line L592 (49.9878, -146.8242) -> (50.4219, -146.6443)
  line L593 (50.4219, -146.6443) -> (50.7946, -146.3582)
  line L594 (50.7946, -146.3582) -> (51.0806, -145.9854)
  line L595 (51.0806, -145.9854) -> (51.2604, -145.5512)
  line L596 (51.2604, -145.5512) -> (51.3217, -145.0853)
  line L597 (27.8041, -144.5752) -> (27.7428, -145.0411)
  line L598 (27.7428, -145.0411) -> (27.8042, -145.5069)
  line L599 (27.8042, -145.5069) -> (27.9841, -145.941)
  line L600 (27.9841, -145.941) -> (28.2702, -146.3138)
  line L601 (28.2702, -146.3138) -> (28.643, -146.5998)
  line L602 (28.643, -146.5998) -> (29.0772, -146.7795)
  line L603 (29.0772, -146.7795) -> (29.5431, -146.8408)
  line L604 (29.5431, -146.8408) -> (30.0089, -146.7794)
  line L605 (30.0089, -146.7794) -> (30.443, -146.5995)
  line L606 (30.443, -146.5995) -> (30.8158, -146.3134)
  line L607 (30.8158, -146.3134) -> (31.1018, -145.9406)
  line L608 (31.1018, -145.9406) -> (31.2815, -145.5064)
  line L609 (31.2815, -145.5064) -> (31.3428, -145.0405)
  line L610 (31.3428, -145.0405) -> (31.2814, -144.5747)
  line L611 (31.2814, -144.5747) -> (31.1015, -144.1406)
  line L612 (31.1015, -144.1406) -> (30.8154, -143.7678)
  line L613 (30.8154, -143.7678) -> (30.4426, -143.4818)
  line L614 (30.4426, -143.4818) -> (30.0084, -143.3021)
  line L615 (30.0084, -143.3021) -> (29.5426, -143.2408)
  line L616 (29.5426, -143.2408) -> (29.0767, -143.3022)
  line L617 (29.0767, -143.3022) -> (28.6426, -143.4821)
  line L618 (28.6426, -143.4821) -> (28.2698, -143.7682)
  line L619 (28.2698, -143.7682) -> (27.9838, -144.141)
  line L620 (27.9838, -144.141) -> (27.8041, -144.5752)
  line L621 (51.2449, 174.5259) -> (51.3062, 174.9918)
  line L622 (51.3062, 174.9918) -> (51.2448, 175.4576)
  line L623 (51.2448, 175.4576) -> (51.0649, 175.8917)
  line L624 (51.0649, 175.8917) -> (50.7788, 176.2645)
  line L625 (50.7788, 176.2645) -> (50.406, 176.5505)
  line L626 (50.406, 176.5505) -> (49.9718, 176.7303)
  line L627 (49.9718, 176.7303) -> (49.506, 176.7915)
  line L628 (49.506, 176.7915) -> (49.0401, 176.7301)
  line L629 (49.0401, 176.7301) -> (48.606, 176.5502)
  line L630 (48.606, 176.5502) -> (48.2332, 176.2641)
  line L631 (48.2332, 176.2641) -> (47.9472, 175.8913)
  line L632 (47.9472, 175.8913) -> (47.7675, 175.4571)
  line L633 (47.7675, 175.4571) -> (47.7062, 174.9913)
  line L634 (47.7062, 174.9913) -> (47.7676, 174.5254)
  line L635 (47.7676, 174.5254) -> (47.9475, 174.0913)
  line L636 (47.9475, 174.0913) -> (48.2336, 173.7185)
  line L637 (48.2336, 173.7185) -> (48.6064, 173.4325)
  line L638 (48.6064, 173.4325) -> (49.0406, 173.2528)
  line L639 (49.0406, 173.2528) -> (49.5065, 173.1915)
  line L640 (49.5065, 173.1915) -> (49.9723, 173.2529)
  line L641 (49.9723, 173.2529) -> (50.4064, 173.4328)
  line L642 (50.4064, 173.4328) -> (50.7792, 173.7189)
  line L643 (50.7792, 173.7189) -> (51.0652, 174.0917)
  line L644 (51.0652, 174.0917) -> (51.2449, 174.5259)
  line L645 (29.5321, 173.1585) -> (29.998, 173.2199)
  line L646 (29.998, 173.2199) -> (30.4321, 173.3998)
  line L647 (30.4321, 173.3998) -> (30.8049, 173.6859)
  line L648 (30.8049, 173.6859) -> (31.0909, 174.0587)
  line L649 (31.0909, 174.0587) -> (31.2706, 174.4929)
  line L650 (31.2706, 174.4929) -> (31.3319, 174.9588)
  line L651 (31.3319, 174.9588) -> (31.2705, 175.4246)
  line L652 (31.2705, 175.4246) -> (31.0906, 175.8587)
  line L653 (31.0906, 175.8587) -> (30.8045, 176.2315)
  line L654 (30.8045, 176.2315) -> (30.4317, 176.5175)
  line L655 (30.4317, 176.5175) -> (29.9975, 176.6972)
  line L656 (29.9975, 176.6972) -> (29.5316, 176.7585)
  line L657 (29.5316, 176.7585) -> (29.0658, 176.6971)
  line L658 (29.0658, 176.6971) -> (28.6317, 176.5172)
  line L659 (28.6317, 176.5172) -> (28.2589, 176.2311)
  line L660 (28.2589, 176.2311) -> (27.9729, 175.8583)
  line L661 (27.9729, 175.8583) -> (27.7931, 175.4241)
  line L662 (27.7931, 175.4241) -> (27.7319, 174.9582)
  line L663 (27.7319, 174.9582) -> (27.7933, 174.4924)
  line L664 (27.7933, 174.4924) -> (27.9732, 174.0583)
  line L665 (27.9732, 174.0583) -> (28.2593, 173.6855)
  line L666 (28.2593, 173.6855) -> (28.6321, 173.3995)
  line L667 (28.6321, 173.3995) -> (29.0663, 173.2198)
  line L668 (29.0663, 173.2198) -> (29.5321, 173.1585)
  line L669 (18.3406, 154.9682) -> (18.2763, 155.4337)
  line L670 (18.2763, 155.4337) -> (18.0936, 155.8666)
  line L671 (18.0936, 155.8666) -> (17.8052, 156.2376)
  line L672 (17.8052, 156.2376) -> (17.4305, 156.5212)
  line L673 (17.4305, 156.5212) -> (16.9953, 156.6982)
  line L674 (16.9953, 156.6982) -> (16.529, 156.7565)
  line L675 (16.529, 156.7565) -> (16.0635, 156.6922)
  line L676 (16.0635, 156.6922) -> (15.6306, 156.5095)
  line L677 (15.6306, 156.5095) -> (15.2596, 156.2211)
  line L678 (15.2596, 156.2211) -> (14.976, 155.8464)
  line L679 (14.976, 155.8464) -> (14.799, 155.4112)
  line L680 (14.799, 155.4112) -> (14.7407, 154.9449)
  line L681 (14.7407, 154.9449) -> (14.805, 154.4794)
  line L682 (14.805, 154.4794) -> (14.9877, 154.0465)
  line L683 (14.9877, 154.0465) -> (15.2761, 153.6756)
  line L684 (15.2761, 153.6756) -> (15.6508, 153.3919)
  line L685 (15.6508, 153.3919) -> (16.0861, 153.2149)
  line L686 (16.0861, 153.2149) -> (16.5523, 153.1566)
  line L687 (16.5523, 153.1566) -> (17.0178, 153.221)
  line L688 (17.0178, 153.221) -> (17.4507, 153.4036)
  line L689 (17.4507, 153.4036) -> (17.8217, 153.692)
  line L690 (17.8217, 153.692) -> (18.1053, 154.0667)
  line L691 (18.1053, 154.0667) -> (18.2823, 154.502)
  line L692 (18.2823, 154.502) -> (18.3406, 154.9682)
  line L693 (18.3279, -0.0318) -> (18.2665, 0.434)
  line L694 (18.2665, 0.434) -> (18.0866, 0.8681)
  line L695 (18.0866, 0.8681) -> (17.8005, 1.2409)
  line L696 (17.8005, 1.2409) -> (17.4277, 1.5269)
  line L697 (17.4277, 1.5269) -> (16.9935, 1.7066)
  line L698 (16.9935, 1.7066) -> (16.5276, 1.7679)
  line L699 (16.5276, 1.7679) -> (16.0618, 1.7065)
  line L700 (16.0618, 1.7065) -> (15.6277, 1.5266)
  line L701 (15.6277, 1.5266) -> (15.2549, 1.2405)
  line L702 (15.2549, 1.2405) -> (14.9689, 0.8677)
  line L703 (14.9689, 0.8677) -> (14.7892, 0.4335)
  line L704 (14.7892, 0.4335) -> (14.7279, -0.0324)
  line L705 (14.7279, -0.0324) -> (14.7893, -0.4982)
  line L706 (14.7893, -0.4982) -> (14.9692, -0.9323)
  line L707 (14.9692, -0.9323) -> (15.2553, -1.3051)
  line L708 (15.2553, -1.3051) -> (15.6281, -1.5911)
  line L709 (15.6281, -1.5911) -> (16.0623, -1.7708)
  line L710 (16.0623, -1.7708) -> (16.5281, -1.8321)
  line L711 (16.5281, -1.8321) -> (16.994, -1.7707)
  line L712 (16.994, -1.7707) -> (17.4281, -1.5908)
  line L713 (17.4281, -1.5908) -> (17.8009, -1.3047)
  line L714 (17.8009, -1.3047) -> (18.0869, -0.9319)
  line L715 (18.0869, -0.9319) -> (18.2666, -0.4977)
  line L716 (18.2666, -0.4977) -> (18.3279, -0.0318)
  line L717 (-270.7214, -148.3819) -> (-270.7214, -139.3819)
  line L718 (-270.7214, -139.3819) -> (-264.2214, -139.3819)
  line L719 (-264.2214, -139.3819) -> (-264.2214, -148.3819)
  line L720 (-264.2214, -148.3819) -> (-270.7214, -148.3819)
  line L721 (-270.7214, -20.6818) -> (-270.7214, -11.6818)
  line L722 (-270.7214, -11.6818) -> (-264.2214, -11.6818)
  line L723 (-264.2214, -11.6818) -> (-264.2214, -20.6818)
  line L724 (-264.2214, -20.6818) -> (-270.7214, -20.6818)
  line L725 (-270.7214, 11.6182) -> (-270.7214, 20.6182)
  line L726 (-270.7214, 20.6182) -> (-264.2214, 20.6182)
  line L727 (-264.2214, 20.6182) -> (-264.2214, 11.6182)
  line L728 (-264.2214, 11.6182) -> (-270.7214, 11.6182)
  line L729 (-270.7214, 134.4109) -> (-270.7214, 143.4109)
  line L730 (-270.7214, 143.4109) -> (-264.2214, 143.4109)
  line L731 (-264.2214, 143.4109) -> (-264.2214, 134.4109)
  line L732 (-264.2214, 134.4109) -> (-270.7214, 134.4109)
  line L733 (-270.7214, 166.7109) -> (-270.7214, 175.7109)
  line L734 (-270.7214, 175.7109) -> (-264.2214, 175.7109)
  line L735 (-264.2214, 175.7109) -> (-264.2214, 166.7109)
  line L736 (-264.2214, 166.7109) -> (-270.7214, 166.7109)
  line L737 (13.2786, -148.3819) -> (13.2786, -139.3819)
  line L738 (13.2786, -139.3819) -> (19.7786, -139.3819)
  line L739 (19.7786, -139.3819) -> (19.7786, -148.3819)
  line L740 (19.7786, -148.3819) -> (13.2786, -148.3819)
  line L741 (13.2786, -20.6818) -> (13.2786, -11.6818)
  line L742 (13.2786, -11.6818) -> (19.7786, -11.6818)
  line L743 (19.7786, -11.6818) -> (19.7786, -20.6818)
  line L744 (19.7786, -20.6818) -> (13.2786, -20.6818)
  line L745 (13.2786, 11.6182) -> (13.2786, 20.6182)
  line L746 (13.2786, 20.6182) -> (19.7786, 20.6182)
  line L747 (19.7786, 20.6182) -> (19.7786, 11.6182)
  line L748 (19.7786, 11.6182) -> (13.2786, 11.6182)
  line L749 (13.2786, 134.4109) -> (13.2786, 143.4109)
  line L750 (13.2786, 143.4109) -> (19.7786, 143.4109)
  line L751 (19.7786, 143.4109) -> (19.7786, 134.4109)
  line L752 (19.7786, 134.4109) -> (13.2786, 134.4109)
  line L753 (13.2786, 166.7109) -> (13.2786, 175.7109)
  line L754 (13.2786, 175.7109) -> (19.7786, 175.7109)
  line L755 (19.7786, 175.7109) -> (19.7786, 166.7109)
  line L756 (19.7786, 166.7109) -> (13.2786, 166.7109)
  line L757 (-285.4136, -171.1313) -> (-286.4489, -170.995)
  line L758 (-286.4489, -170.995) -> (-294.4449, -170.995)
  line L759 (-294.4449, -170.995) -> (-295.4802, -171.1313)
  line L760 (-295.4802, -171.1313) -> (-296.4449, -171.5309)
  line L761 (-296.4449, -171.5309) -> (-297.2733, -172.1666)
  line L762 (-297.2733, -172.1666) -> (-297.909, -172.995)
  line L763 (-297.909, -172.995) -> (-298.3086, -173.9597)
  line L764 (-298.3086, -173.9597) -> (-298.4449, -174.995)
  line L765 (-298.4449, -174.995) -> (-298.3086, -176.0303)
  line L766 (-298.3086, -176.0303) -> (-297.909, -176.995)
  line L767 (-297.909, -176.995) -> (-297.2733, -177.8234)
  line L768 (-297.2733, -177.8234) -> (-296.4449, -178.4591)
  line L769 (-296.4449, -178.4591) -> (-295.4802, -178.8587)
  line L770 (-295.4802, -178.8587) -> (-294.4449, -178.995)
  line L771 (-294.4449, -178.995) -> (-286.3821, -178.995)
  line L772 (-286.3821, -178.995) -> (-285.4136, -178.8587)
  line L773 (-285.4136, -178.8587) -> (-284.4489, -178.4591)
  line L774 (-284.4489, -178.4591) -> (-283.6205, -177.8234)
  line L775 (-283.6205, -177.8234) -> (-282.9848, -176.995)
  line L776 (-282.9848, -176.995) -> (-282.5852, -176.0303)
  line L777 (-282.5852, -176.0303) -> (-282.4489, -174.995)
  line L778 (-282.4489, -174.995) -> (-282.5852, -173.9597)
  line L779 (-282.5852, -173.9597) -> (-282.9848, -172.995)
  line L780 (-282.9848, -172.995) -> (-283.6205, -172.1666)
  line L781 (-283.6205, -172.1666) -> (-284.4489, -171.5309)
  line L782 (-284.4489, -171.5309) -> (-285.4136, -171.1313)
  line L783 (44.1238, -171.1313) -> (43.0886, -170.995)
  line L784 (43.0886, -170.995) -> (35.0926, -170.995)
  line L785 (35.0926, -170.995) -> (34.0573, -171.1313)
  line L786 (34.0573, -171.1313) -> (33.0926, -171.5309)
  line L787 (33.0926, -171.5309) -> (32.2642, -172.1666)
  line L788 (32.2642, -172.1666) -> (31.6285, -172.995)
  line L789 (31.6285, -172.995) -> (31.2289, -173.9597)
  line L790 (31.2289, -173.9597) -> (31.0926, -174.995)
  line L791 (31.0926, -174.995) -> (31.2289, -176.0303)
  line L792 (31.2289, -176.0303) -> (31.6285, -176.995)
  line L793 (31.6285, -176.995) -> (32.2642, -177.8234)
  line L794 (32.2642, -177.8234) -> (33.0926, -178.4591)
  line L795 (33.0926, -178.4591) -> (34.0573, -178.8587)
  line L796 (34.0573, -178.8587) -> (35.0926, -178.995)
  line L797 (35.0926, -178.995) -> (43.1554, -178.995)
  line L798 (43.1554, -178.995) -> (44.1238, -178.8587)
  line L799 (44.1238, -178.8587) -> (45.0886, -178.4591)
  line L800 (45.0886, -178.4591) -> (45.917, -177.8234)
  line L801 (45.917, -177.8234) -> (46.5527, -176.995)
  line L802 (46.5527, -176.995) -> (46.9523, -176.0303)
  line L803 (46.9523, -176.0303) -> (47.0886, -174.995)
  line L804 (47.0886, -174.995) -> (46.9523, -173.9597)
  line L805 (46.9523, -173.9597) -> (46.5527, -172.995)
  line L806 (46.5527, -172.995) -> (45.917, -172.1666)
  line L807 (45.917, -172.1666) -> (45.0886, -171.5309)
  line L808 (45.0886, -171.5309) -> (44.1238, -171.1313)
  line L809 (39.2489, -178.995) -> (39.5286, -179.0318)
  line L810 (39.5286, -179.0318) -> (39.8083, -178.995)
  line L811 (-30.4714, -145.0318) -> (-35.4714, -150.0318)
  line L812 (-35.4714, -150.0318) -> (-35.4714, -165.0974)
  line L813 (-35.4714, -165.0974) -> (-35.6334, -166.3282)
  line L814 (-35.6334, -166.3282) -> (-36.1338, -167.5361)
  line L815 (-36.1338, -167.5361) -> (-36.9297, -168.5735)
  line L816 (-36.9297, -168.5735) -> (-37.9671, -169.3694)
  line L817 (-37.9671, -169.3694) -> (-39.1751, -169.8698)
  line L818 (-39.1751, -169.8698) -> (-40.4714, -170.0405)
  line L819 (-40.4714, -170.0405) -> (-41.7677, -169.8698)
  line L820 (-41.7677, -169.8698) -> (-42.9757, -169.3694)
  line L821 (-42.9757, -169.3694) -> (-44.013, -168.5735)
  line L822 (-44.013, -168.5735) -> (-44.809, -167.5361)
  line L823 (-44.809, -167.5361) -> (-45.3093, -166.3282)
  line L824 (-45.3093, -166.3282) -> (-45.4714, -165.0974)
  line L825 (-45.4714, -165.0974) -> (-45.4714, -150.0318)
  line L826 (-45.4714, -150.0318) -> (-50.4714, -145.0318)
  line L827 (-50.4714, -145.0318) -> (-95.4714, -145.0318)
  line L828 (-95.4714, -145.0318) -> (-120.4714, -170.0318)
  line L829 (-120.4714, -170.0318) -> (-130.4714, -170.0318)
  line L830 (-130.4714, -170.0318) -> (-155.4714, -145.0318)
  line L831 (-155.4714, -145.0318) -> (-200.4714, -145.0318)
  line L832 (-200.4714, -145.0318) -> (-205.4714, -150.0318)
  line L833 (-205.4714, -150.0318) -> (-205.4714, -165.0974)
  line L834 (-205.4714, -165.0974) -> (-205.6334, -166.3282)
  line L835 (-205.6334, -166.3282) -> (-206.1338, -167.5361)
  line L836 (-206.1338, -167.5361) -> (-206.9297, -168.5735)
  line L837 (-206.9297, -168.5735) -> (-207.9671, -169.3694)
  line L838 (-207.9671, -169.3694) -> (-209.175, -169.8698)
  line L839 (-209.175, -169.8698) -> (-210.4714, -170.0405)
  line L840 (-210.4714, -170.0405) -> (-211.7677, -169.8698)
  line L841 (-211.7677, -169.8698) -> (-212.9757, -169.3694)
  line L842 (-212.9757, -169.3694) -> (-214.013, -168.5735)
  line L843 (-214.013, -168.5735) -> (-214.809, -167.5361)
  line L844 (-214.809, -167.5361) -> (-215.3093, -166.3282)
  line L845 (-215.3093, -166.3282) -> (-215.4714, -165.0974)
  line L846 (-215.4714, -165.0974) -> (-215.4714, -150.0318)
  line L847 (-215.4714, -150.0318) -> (-220.4714, -145.0318)
  line L848 (-220.4714, -145.0318) -> (-250.4714, -145.0318)
  line L849 (-250.4714, -145.0318) -> (-255.4714, -140.0318)
  line L850 (-255.4714, -140.0318) -> (-255.4714, 139.9681)
  line L851 (-255.4714, 139.9681) -> (-250.4714, 144.9681)
  line L852 (-250.4714, 144.9681) -> (-0.4714, 144.9681)